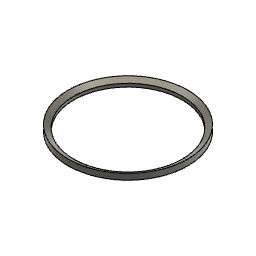
Wheel Spacer (Autodesk Fusion 360 design; units mm, degrees)
Autodesk Fusion 360 part; units mm, degrees
sketch "Sketch1" plane through (0, 0, 0) normal (0, 0, 1) x (1, 0, 0)
  line L0 (0, 0) -> (5, 0)
  line L1 (0, 0) -> (0, 3)
  line L2 (5, 0) -> (5, 5.5)
  line L3 (0, 3) -> (5, 5.5)
  dimension "d1" = 5
  dimension "d2" = 3
  dimension "d3" = 5.5
  constraint coincident L0.start L1.start
  constraint horizontal L0
  constraint perpendicular L0 L1
  constraint perpendicular L0 L2
  measures "d1" distance of L0.start L0.end
  measures "d2" distance of L0.start L1.end
  measures "d3" distance of L0.end L2.end
sketch "Sketch2" plane through (0, 0, 0) normal (0, 1, 0) x (1, 0, 0)
  line L0 (0, 0) -> (-50.25, 0)
  circle A0 centre (-50.25, 0) radius 2.5
  dimension "d4" = 50.25
  dimension "d6" = 5
  constraint coincident L0.start origin
  constraint horizontal L0
  constraint coincident L0.end A0.centre
  measures "d4" distance of L0.start L0.end
  measures "d6" diameter of A0
extrude "Extrude1" add sketch "Sketch2" along normal blind 100 makes body 1
revolve "Revolve1" add sketch "Sketch1" angle 360 about axis through (-50.25, 0, 0) along (0, -1, 0) separate body makes body 2
delete_body "RemoveBody1" bodies 1
equation "d3 = 7.5 mm - 2 mm"
equation "d4 = ( 100.5 / 2 ) * 1 mm"
